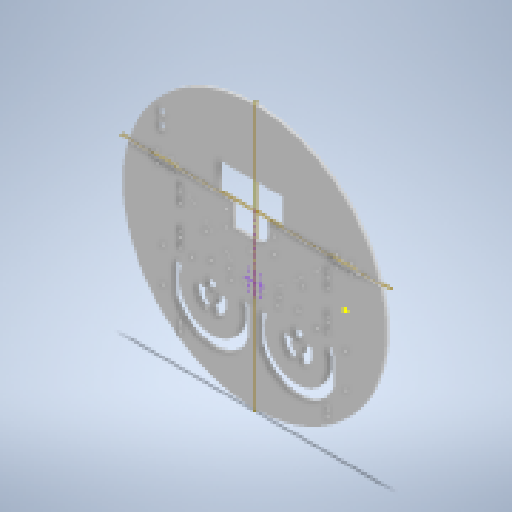
# Autodesk Inventor part: Деталь1
Saved by Autodesk Inventor 2023.2 (Build 272271030, 271C)
## iProperties
Created: 2024-01-26
Part Number: Деталь1
Material: Типовые
Document SubType Name: Modeling
Designer: I9232
Density: 1 g/cm^3
Appearance: По умолчанию
Author: I9232
Autodesk Inventor part; units mm, degrees
ref_plane "YZ Plane" through (0, 0, 0) normal (1, 0, 0) x (0, 1, 0)
ref_plane "XY Plane" through (0, 0, 0) normal (0, 0, 1) x (1, 0, 0)
sketch "Эскиз1" plane through (0, 0, 0) normal (0, 0, 1) x (1, 0, 0)
  circle A0 centre (-95.6307, 0) radius 137.5
  point P0 (0, 0)
  dimension "d61" = 275
  constraints: 1 centre point, 1 other
  measures "d61" diameter of A0
extrude "Выдавливание1" add sketch "Эскиз1" along normal blind 3
sketch "Эскиз5" plane through (0, 0, 3) normal (0, 0, 1) x (1, 0, 0)
  circle A0 centre (-191.4705, -72.9366) radius 1.5
  circle A1 centre (-191.4705, -37.0634) radius 1.5
  circle A2 centre (0, -37.0634) radius 1.5
  circle A3 centre (0, -72.9366) radius 1.5
  circle A4 centre (-30.8327, -32.3517) radius 1.5 projected
  circle A5 centre (-50.2499, -25.7302) radius 1.5 projected
  circle A6 centre (-70.9883, -32.7537) radius 1.5 projected
  circle A7 centre (-120.4823, -32.7537) radius 1.5 projected
  circle A8 centre (-141.2206, -25.7302) radius 1.5 projected
  circle A9 centre (-160.6378, -32.3517) radius 1.5 projected
  arc A10 (-12.7161, -49.3219) -> (-16.1637, -41.7649) centre (-51.5496, -62.4733) ccw projected
  line L0 (-12.7161, -49.3219) -> (-13.1664, -76.8861) projected
  arc A11 (-89.9328, -76.8861) -> (-13.1664, -76.8861) centre (-51.5496, -62.4733) ccw projected
  line L1 (-89.9328, -76.8861) -> (-90.3831, -49.3219) projected
  arc A12 (-88.8603, -45.4758) -> (-90.3831, -49.3219) centre (-51.5496, -62.4733) ccw projected
  line L2 (-88.8603, -45.4758) -> (-82.9355, -45.4758) projected
  arc A13 (-82.9355, -45.4758) -> (-20.1637, -46.3085) centre (-51.725, -59.1185) ccw projected
  line L3 (-20.1637, -46.3085) -> (-16.1637, -41.7649) projected
  line L4 (-178.9659, -76.8861) -> (-179.4162, -49.3219) projected
  arc A14 (-175.9686, -41.7649) -> (-179.4162, -49.3219) centre (-140.5827, -62.4733) ccw projected
  line L5 (-175.9686, -41.7649) -> (-171.9686, -46.3085) projected
  arc A15 (-171.9686, -46.3085) -> (-109.1968, -46.3085) centre (-140.5827, -59.1724) ccw projected
  line L6 (-109.1968, -46.3085) -> (-103.2721, -45.4758) projected
  arc A16 (-101.7492, -49.3219) -> (-103.2721, -45.4758) centre (-140.5827, -62.4733) ccw projected
  line L7 (-101.7492, -49.3219) -> (-102.1995, -76.8861) projected
  arc A17 (-178.9659, -76.8861) -> (-102.1995, -76.8861) centre (-140.5827, -62.4733) ccw projected
  arc A18 (-45.6461, -44.0105) -> (-55.6209, -44) centre (-50.6489, -58.6809) ccw projected
  line L8 (-45.6461, -44.0105) -> (-47.4855, -52.1853) projected
  arc A19 (-47.4855, -52.1853) -> (-53.8449, -52.3024) centre (-50.5504, -58.4786) ccw projected
  line L9 (-53.8449, -52.3024) -> (-55.6209, -44) projected
  line L10 (-135.8496, -44) -> (-137.6256, -52.3024) projected
  arc A20 (-137.6256, -52.3024) -> (-143.985, -52.1853) centre (-140.9201, -58.4786) ccw projected
  line L11 (-143.985, -52.1853) -> (-145.8244, -44.0105) projected
  arc A21 (-135.8496, -44) -> (-145.8244, -44.0105) centre (-140.8216, -58.6809) ccw projected
  arc A22 (-135.8665, -73.3675) -> (-126.822, -52.0281) centre (-140.8216, -58.6809) ccw projected
  line L12 (-135.8665, -73.3675) -> (-138.9215, -65.1872) projected
  arc A23 (-138.9215, -65.1872) -> (-135.0144, -54.7207) centre (-140.9201, -58.4786) ccw projected
  line L13 (-135.0144, -54.7207) -> (-126.822, -52.0281) projected
  arc A24 (-64.6485, -52.0281) -> (-55.604, -73.3675) centre (-50.6489, -58.6809) ccw projected
  line L14 (-64.6485, -52.0281) -> (-56.4561, -54.7207) projected
  arc A25 (-56.4561, -54.7207) -> (-52.549, -65.1872) centre (-50.5504, -58.4786) ccw projected
  line L15 (-52.549, -65.1872) -> (-55.604, -73.3675) projected
  arc A26 (-45.6939, -73.3676) -> (-36.6645, -51.9961) centre (-50.6489, -58.6809) ccw projected
  line L16 (-45.6939, -73.3676) -> (-48.7266, -65.2369) projected
  arc A27 (-48.7266, -65.2369) -> (-44.6776, -54.6694) centre (-50.5504, -58.4786) ccw projected
  line L17 (-44.6776, -54.6694) -> (-36.6645, -51.9961) projected
  arc A28 (-146.793, -54.6694) -> (-142.7439, -65.2369) centre (-140.9201, -58.4786) ccw projected
  line L18 (-142.7439, -65.2369) -> (-145.7766, -73.3676) projected
  arc A29 (-154.806, -51.9961) -> (-145.7766, -73.3676) centre (-140.8216, -58.6809) ccw projected
  line L19 (-154.806, -51.9961) -> (-146.793, -54.6694) projected
  dimension "d94" = 3
  dimension "d95" = 191.4705
  constraints: 4 centre point, 3 equal radius
  measures "d94" diameter of A3
  measures "d95" distance of A3.centre A0.centre
extrude "Выдавливание5" cut sketch "Эскиз5" against normal blind 3
sketch "Эскиз11" plane through (-95.6307, 0, 3) normal (0, 0, 1) x (1, 0, 0)
  line L0 (-6.5688, -36.8861) -> (-6.1185, -9.3219) construction
  line L1 (-6.3437, -23.104) -> (5.4727, -23.104) construction
  line L2 (5.6979, -36.8861) -> (5.2476, -9.3219) construction
  line L3 (-0.4355, 43.8357) -> (-0.4355, -36.6138) construction
  point P0 (95.6307, 0)
  point P1 (-0.4355, -23.104)
  constraints: 8 end point, 3 midpoint, 1 point on line, 1 vertical
ref_plane "Плоскость центральной симметрии" through (-96.0662, 43.8357, 3) normal (-1, 0, 0) x (0, -1, 0)
sketch "Эскиз8" plane through (0, 0, 3) normal (0, 0, 1) x (1, 0, 0)
  circle A0 centre (-197.0662, 34.25) radius 1.25
  circle A1 centre (-183.0662, 34.25) radius 1.25
  line L0 (-96.0662, -192.5) -> (-96.0662, 192.5) projected
  line L1 (-183.0662, 34.25) -> (-197.0662, 34.25) construction
  circle A2 centre (-183.0662, 44.75) radius 1.25
  circle A3 centre (-197.0662, 44.75) radius 1.25
  circle A4 centre (4.9338, 34.25) radius 1.25
  circle A5 centre (-9.0662, 34.25) radius 1.25
  line L2 (-9.0662, 34.25) -> (4.9338, 34.25) construction
  circle A6 centre (-9.0662, 44.75) radius 1.25
  circle A7 centre (4.9338, 44.75) radius 1.25
  line L3 (-183.0662, 34.25) -> (-183.0662, 44.75) construction
  line L4 (-183.0662, 39.5) -> (-192.8856, 39.5) construction
  line L5 (-197.0662, 44.75) -> (-197.0662, 34.25) construction
  point P0 (0, 0)
  dimension "d23" = 87
  dimension "d24" = 14
  dimension "d26" = 2.5
  dimension "d29" = 10.5
  dimension "d96" = 39.5
  constraints: 10 end point, 8 centre point, 4 symmetric about line, 3 vertical, 2 horizontal, 1 equal radius, 1 midpoint, 8 other
  measures "d23" distance from line of L1.start L0
  measures "d24" distance of L1.end L1.start
  measures "d26" diameter of A1
  measures "d29" distance of L1.start L3.end
  measures "d96" distance from line of L4 point (0, 0)
extrude "Выдавливание8" cut sketch "Эскиз8" against normal blind 3
sketch "Эскиз9" plane through (0, 0, 3) normal (0, 0, 1) x (1, 0, 0)
  point P0 (0, 0)
ref_plane "РабПлоскость2" through (0, 40, 0) normal (0, 1, 0) x (-1, 0, 0)
split body "Разделение2" result two bodies by plane through (0, 40, 0) normal (0, 1, 0) first body at (-95.921, 75.6667, 0.5)
sketch "Эскиз3" plane through (-95.6307, 0, 3) normal (0, 0, 1) x (1, 0, 0)
  circle A0 centre (0, 0) radius 137.5 projected
  line L0 (131.8531, 39) -> (-131.8531, 39)
  line L1 (131.245, 41) -> (-131.245, 41)
  arc A1 (-131.245, 41) -> (-131.8531, 39) centre (0, 0) ccw
  arc A2 (131.8531, 39) -> (131.245, 41) centre (9.2386, 2.8092) ccw
  line L2 (-192.5, 40) -> (192.5, 40) projected
  line L3 (-112.9264, 39) -> (-112.9264, 41) construction
  line L4 (131.5532, 40) -> (-131.5532, 40) projected
  point P0 (95.6307, 0)
  point P1 (-112.9264, 40)
  dimension "d63" = 2
  constraints: 8 point on circle, 6 end point, 3 point on line, 2 centre point, 1 concentric, 1 horizontal, 1 midpoint, 1 parallel, 1 perpendicular
  measures "d63" distance between parallel lines of L1 L0
extrude "Выдавливание3" cut sketch "Эскиз3" against normal blind 3 contours L0 A0 L2 | L2 A0 L1 bodies 2 3
sketch "Эскиз12" plane through (0, 0, 3) normal (0, 0, 1) x (1, 0, 0)
  line L0 (-171.3841, -10.2204) -> (-174.3841, -10.2204)
  line L1 (-174.3841, -10.2204) -> (-174.3841, -17.2204)
  line L2 (-174.3841, -17.2204) -> (-171.3841, -17.2204)
  line L3 (-171.3841, -17.2204) -> (-171.3841, -10.2204)
  line L4 (-171.3841, 15.777) -> (-174.3841, 15.777)
  line L5 (-174.3841, 15.777) -> (-174.3841, 8.777)
  line L6 (-174.3841, 8.777) -> (-171.3841, 8.777)
  line L7 (-171.3841, 8.777) -> (-171.3841, 15.777)
  line L8 (-171.3841, 29.777) -> (-174.3841, 29.777)
  line L9 (-174.3841, 29.777) -> (-174.3841, 22.777)
  line L10 (-174.3841, 22.777) -> (-171.3841, 22.777)
  line L11 (-171.3841, 22.777) -> (-171.3841, 29.777)
  line L12 (-174.3841, -108.1269) -> (-171.3841, -108.1269)
  line L13 (-171.3841, -108.1269) -> (-171.3841, -104.1269)
  line L14 (-171.3841, -104.1269) -> (-174.3841, -104.1269)
  line L15 (-174.3841, -104.1269) -> (-174.3841, -108.1269)
  line L16 (-174.3841, -99.1269) -> (-171.3841, -99.1269)
  line L17 (-171.3841, -99.1269) -> (-171.3841, -95.1269)
  line L18 (-171.3841, -95.1269) -> (-174.3841, -95.1269)
  line L19 (-174.3841, -95.1269) -> (-174.3841, -99.1269)
  line L20 (-96.0662, -192.5) -> (-96.0662, 192.5) construction
  line L21 (-171.3841, -24.2204) -> (-174.3841, -24.2204)
  line L22 (-174.3841, -24.2204) -> (-174.3841, -31.2204)
  line L23 (-174.3841, -31.2204) -> (-171.3841, -31.2204)
  line L24 (-171.3841, -31.2204) -> (-171.3841, -24.2204)
  line L25 (-20.7483, -10.2204) -> (-17.7483, -10.2204)
  line L26 (-17.7483, -10.2204) -> (-17.7483, -17.2204)
  line L27 (-17.7483, -17.2204) -> (-20.7483, -17.2204)
  line L28 (-20.7483, -17.2204) -> (-20.7483, -10.2204)
  line L29 (-20.7483, 15.777) -> (-17.7483, 15.777)
  line L30 (-17.7483, 15.777) -> (-17.7483, 8.777)
  line L31 (-17.7483, 8.777) -> (-20.7483, 8.777)
  line L32 (-20.7483, 8.777) -> (-20.7483, 15.777)
  line L33 (-20.7483, 29.777) -> (-17.7483, 29.777)
  line L34 (-17.7483, 29.777) -> (-17.7483, 22.777)
  line L35 (-17.7483, 22.777) -> (-20.7483, 22.777)
  line L36 (-20.7483, 22.777) -> (-20.7483, 29.777)
  line L37 (-17.7483, -108.1269) -> (-20.7483, -108.1269)
  line L38 (-20.7483, -108.1269) -> (-20.7483, -104.1269)
  line L39 (-20.7483, -104.1269) -> (-17.7483, -104.1269)
  line L40 (-17.7483, -104.1269) -> (-17.7483, -108.1269)
  line L41 (-17.7483, -99.1269) -> (-20.7483, -99.1269)
  line L42 (-20.7483, -99.1269) -> (-20.7483, -95.1269)
  line L43 (-20.7483, -95.1269) -> (-17.7483, -95.1269)
  line L44 (-17.7483, -95.1269) -> (-17.7483, -99.1269)
  line L45 (-20.7483, -24.2204) -> (-17.7483, -24.2204)
  line L46 (-17.7483, -24.2204) -> (-17.7483, -31.2204)
  line L47 (-17.7483, -31.2204) -> (-20.7483, -31.2204)
  line L48 (-20.7483, -31.2204) -> (-20.7483, -24.2204)
  circle A0 centre (-172.8841, -20.7204) radius 1.5
  circle A1 centre (-172.8841, -101.6269) radius 1.5
  circle A2 centre (-172.8841, 19.277) radius 1.5
  line L49 (-20.7483, -24.2204) -> (-17.7483, -24.2204)
  circle A3 centre (-19.2483, -20.7204) radius 1.5
  circle A4 centre (-19.2483, -101.6269) radius 1.5
  circle A5 centre (-19.2483, 19.277) radius 1.5
  point P0 (-172.8841, -99.1269)
  point P1 (-172.8841, -17.2204)
  point P2 (-172.8841, 22.777)
  dimension "d74" = 3
  dimension "d75" = 2.5
  dimension "d76" = 3.5
  dimension "d77" = 3.5
  constraints: 98 end point, 27 symmetric about line, 6 centre point, 3 midpoint, 2 equal radius, 3 other
  measures "d74" diameter of A0
  measures "d75" distance of point (-172.884, -99.127) A1.centre
  measures "d76" distance of point (-172.884, -17.22) A0.centre
  measures "d77" distance of point (-172.884, 22.777) A2.centre
extrude "Выдавливание10" cut sketch "Эскиз12" against normal through all bodies 3
sketch "Эскиз13" plane through (0, 0, 0) normal (0, 0, -1) x (-1, 0, 0)
  line L0 (196.3841, 65.7571) -> (190.3841, 65.7571) construction
  line L1 (190.3841, 65.7571) -> (190.3841, 85.7571) construction
  line L2 (190.3841, 85.7571) -> (196.3841, 85.7571) construction
  line L3 (196.3841, 85.7571) -> (196.3841, 65.7571) construction
  line L4 (196.3841, 65.7571) -> (190.3841, 65.7571)
  line L5 (190.3841, 65.7571) -> (190.3841, 72.7571)
  line L6 (190.3841, 72.7571) -> (196.3841, 72.7571)
  line L7 (196.3841, 72.7571) -> (196.3841, 65.7571)
  line L8 (196.3841, 75.7571) -> (190.3841, 75.7571) construction
  line L9 (196.3841, 85.7571) -> (190.3841, 85.7571) construction
  line L10 (196.3841, 85.7571) -> (190.3841, 85.7571)
  line L11 (190.3841, 85.7571) -> (190.3841, 78.7571)
  line L12 (190.3841, 78.7571) -> (196.3841, 78.7571)
  line L13 (196.3841, 78.7571) -> (196.3841, 85.7571)
  line L14 (149.3841, 76.0844) -> (149.3841, 68.5395) projected
  line L15 (193.3841, 78.7571) -> (193.3841, 72.7571) construction
  circle A0 centre (193.3841, 75.7571) radius 1.5
  line L16 (190.3841, 61.9127) -> (190.3841, 81.7469) projected
  point P0 (0, 0)
  point P1 (190.3841, 82.2571)
  dimension "d37" = 6
  dimension "d38" = 20
  dimension "d39" = 7
  dimension "d43" = 3
  dimension "d66" = 0
  constraints: 30 end point, 6 midpoint, 4 parallel, 4 symmetric about line, 2 horizontal, 2 perpendicular, 1 centre point, 1 point on line
  measures "d37" distance of L8.start L8.end
  measures "d38" distance of L2.end L0.start
  measures "d39" distance between parallel lines of L0 L6
  measures "d43" diameter of A0
  measures "d66" distance from line of L16 point (190.384, 82.257)
extrude "Выдавливание11" cut sketch "Эскиз13" against normal through all bodies 2
sketch "Эскиз16" plane through (0, 0, 3) normal (0, 0, 1) x (1, 0, 0)
  line L0 (-227.4838, 39) -> (36.2225, 39) projected
  line L1 (-96.0662, 39) -> (-96.0662, 41)
  line L2 (35.6143, 41) -> (-226.8757, 41) projected
  arc A0 (-96.0662, 15.3364) -> (-81.5178, 24.1698) centre (-94.6991, 29.482) ccw
  line L3 (-81.5178, 24.1698) -> (-81.5178, 39)
  line L4 (36.2225, 39) -> (-227.4838, 39) projected
  line L5 (-117.5429, 39) -> (-117.5429, 15.3364)
  arc A1 (-74.5894, 41) -> (-117.5429, 39) centre (-96.0662, 40) ccw
  line L6 (-96.0662, 15.3364) -> (-117.5429, 15.3364)
  point P0 (0, 0)
  point P1 (-117.5429, 41)
  constraints: 8 end point, 5 point on line, 4 point on circle, 3 perpendicular, 2 centre point, 1 midpoint
extrude "Выдавливание13" cut sketch "Эскиз16" against normal blind 3 contours L0 L3 A0 L6 L5 | A1 L2 bodies 2 3
sketch "Эскиз17" plane through (0, 0, 3) normal (0, 0, 1) x (1, 0, 0)
  circle A0 centre (-75.0461, 12) radius 1.25 projected
  circle A1 centre (-75.0662, 28.5) radius 1.25 projected
  circle A2 centre (-100.0461, 3.5) radius 1.25 projected
  circle A3 centre (-125.0461, 12) radius 1.25 projected
  circle A4 centre (-125.0662, 28.5) radius 1.25 projected
  point P0 (0, 0)
extrude "Выдавливание14" cut sketch "Эскиз17" against normal blind 3 bodies 3
sketch "Эскиз19" plane through (0, 0, 3) normal (0, 0, 1) x (1, 0, 0)
  circle A0 centre (-75.0461, 12) radius 1.25 projected
  circle A1 centre (-125.0461, 12) radius 1.25 projected
  circle A2 centre (-75.0662, 28.5) radius 1.25 projected
  circle A3 centre (-100.0461, 3.5) radius 1.25 projected
  circle A4 centre (-125.0662, 28.5) radius 1.25 projected
  arc A5 (-68.8662, 60) -> (-73.8662, 65) centre (-73.8662, 60) ccw projected
  arc A6 (-73.8662, -5) -> (-68.8662, 0) centre (-73.8662, 0) ccw projected
  line L0 (-73.8662, -5) -> (-124.2662, -5) projected
  line L1 (-131.2662, 2) -> (-131.2662, 60) projected
  arc A7 (-126.2662, 65) -> (-131.2662, 60) centre (-126.2662, 60) ccw projected
  line L2 (-126.2662, 65) -> (-108.2662, 65) projected
  line L3 (-116.2662, 50) -> (-116.2662, 21.4) projected
  line L4 (-108.2662, 10) -> (-83.8662, 10) projected
  line L5 (-83.8662, 10) -> (-83.8662, 60) projected
  arc A8 (-78.8662, 65) -> (-83.8662, 60) centre (-78.8662, 60) ccw projected
  line L6 (-78.8662, 65) -> (-73.8662, 65) projected
  line L7 (-74.5894, 41) -> (35.6143, 41) projected
  line L8 (-66.8662, 41) -> (-84.8662, 41)
  line L9 (-84.8662, 41) -> (-84.8662, 69)
  line L10 (-84.8662, 69) -> (-66.8662, 69)
  line L11 (-66.8662, 69) -> (-66.8662, 41)
  line L12 (-226.8757, 41) -> (-117.5429, 41) projected
  line L13 (-133.2662, 41) -> (-115.2662, 41)
  line L14 (-115.2662, 41) -> (-115.2662, 69)
  line L15 (-115.2662, 69) -> (-133.2662, 69)
  line L16 (-133.2662, 69) -> (-133.2662, 41)
  line L17 (-116.2662, 21.4) -> (-108.2662, 21.4) projected
  line L18 (-108.2662, 21.4) -> (-108.2662, 10) projected
  line L19 (-108.2662, 65) -> (-108.2662, 50) projected
  line L20 (-108.2662, 50) -> (-116.2662, 50) projected
  line L21 (-84.8662, 69) -> (-115.2662, 69)
  arc A9 (-131.2662, 2) -> (-124.2662, -5) centre (-124.2662, 2) ccw projected
  line L22 (-68.8662, 60) -> (-68.8662, 0) projected
  point P0 (0, 0)
  point P1 (-74.5894, 41)
  point P2 (-83.8662, 41)
  point P3 (-116.0662, 41)
  point P4 (-74.0662, 60)
  point P5 (-74.0662, 0)
  point P6 (-115.2662, 65)
  point P7 (-131.2662, 41)
  point P8 (-74.0662, 60)
  point P9 (-74.0662, 0)
  point P10 (-115.2662, 50)
  point P11 (-74.0662, 60)
  point P12 (-74.0662, 0)
  point P13 (-116.2662, 41)
  point P14 (-74.0662, 60)
  point P15 (-74.0662, 0)
  point P16 (-74.0662, 60)
  point P17 (-74.0662, 0)
  point P18 (-74.0662, 60)
  point P19 (-74.0662, 0)
  dimension "d53" = 28
  dimension "d54" = 28
  dimension "d57" = 1
  dimension "d58" = 1
  dimension "d64" = 18
  dimension "d65" = 18
  constraints: 18 end point, 4 parallel, 3 perpendicular, 3 point on line, 2 horizontal
  measures "d53" distance of L10.end L8.start
  measures "d54" distance of L15.end L13.start
  measures "d57" distance between parallel lines of L9 L5
  measures "d58" distance between parallel lines of L3 L14
  measures "d64" distance of L14.end L15.end
  measures "d65" distance of L9.end L10.end
extrude "Выдавливание15" cut sketch "Эскиз19" against normal blind 3 contours A0 | A1 | A2 | A3 | A4 | L22 L7 L8 L5 A8 L6 A5 | A5 L6 A8 L5 L8 L9 L10 L11 L7 L22 | L22 A6 L0 A9 L1 L12 L13 L3 L17 L18 L4 L5 L8 L7 | L5 L4 L18 L17 L3 L13 L14 L20 L19 L2 L21 L9 L8 | L14 L2 A7 L1 L12 L16 L15 | L14 L20 L3 L13 L12 L1 A7 L2 | L2 L19 L20 L14 | L14 L13 L3 L20 bodies 2
sketch "Эскиз20" plane through (0, 0, 3) normal (0, 0, 1) x (1, 0, 0)
  circle A0 centre (-147.1535, -2.0082) radius 1.45 projected
  circle A1 centre (-121.6186, -23.4345) radius 1.45 projected
  circle A2 centre (-96.0662, -40.2976) radius 1.45 projected
  circle A3 centre (-70.5137, -23.4345) radius 1.45 projected
  circle A4 centre (-44.9789, -2.0082) radius 1.45 projected
  point P0 (0, 0)
extrude "Выдавливание16" cut sketch "Эскиз20" against normal blind 3 bodies 2 3
sketch "Эскиз21" plane through (0, 0, 0) normal (0, 0, -1) x (-1, 0, 0)
  line L0 (147.5387, 7.4529) -> (137.5802, -0.9033) projected
  line L1 (147.5387, 7.4529) -> (147.3459, 7.6827) projected
  line L2 (147.3459, 7.6827) -> (137.3873, -0.6735) projected
  line L3 (137.5802, -0.9033) -> (137.3873, -0.6735) projected
  line L4 (166.8431, 23.6512) -> (156.8845, 15.2949) projected
  line L5 (166.8431, 23.6512) -> (166.6502, 23.881) projected
  line L6 (166.6502, 23.881) -> (156.6917, 15.5247) projected
  line L7 (156.8845, 15.2949) -> (156.6917, 15.5247) projected
  line L8 (128.2344, -8.7453) -> (118.2759, -17.1016) projected
  line L9 (128.2344, -8.7453) -> (128.0416, -8.5155) projected
  line L10 (128.0416, -8.5155) -> (118.083, -16.8718) projected
  line L11 (118.2759, -17.1016) -> (118.083, -16.8718) projected
  line L12 (108.9301, -24.9436) -> (98.9715, -33.2998) projected
  line L13 (108.9301, -24.9436) -> (108.7373, -24.7138) projected
  line L14 (108.7373, -24.7138) -> (98.7787, -33.07) projected
  line L15 (98.9715, -33.2998) -> (98.7787, -33.07) projected
  line L16 (83.2022, -24.9436) -> (93.1608, -33.2998) projected
  line L17 (93.1608, -33.2998) -> (93.3536, -33.07) projected
  line L18 (83.395, -24.7138) -> (93.3536, -33.07) projected
  line L19 (83.2022, -24.9436) -> (83.395, -24.7138) projected
  line L20 (63.8979, -8.7453) -> (73.8565, -17.1016) projected
  line L21 (73.8565, -17.1016) -> (74.0493, -16.8718) projected
  line L22 (64.0907, -8.5155) -> (74.0493, -16.8718) projected
  line L23 (63.8979, -8.7453) -> (64.0907, -8.5155) projected
  line L24 (44.5936, 7.4529) -> (54.5521, -0.9033) projected
  line L25 (54.5521, -0.9033) -> (54.745, -0.6735) projected
  line L26 (44.7864, 7.6827) -> (54.745, -0.6735) projected
  line L27 (44.5936, 7.4529) -> (44.7864, 7.6827) projected
  line L28 (25.2892, 23.6512) -> (35.2478, 15.2949) projected
  line L29 (35.2478, 15.2949) -> (35.4407, 15.5247) projected
  line L30 (25.4821, 23.881) -> (35.4407, 15.5247) projected
  line L31 (25.2892, 23.6512) -> (25.4821, 23.881) projected
  line L32 (21.459, 43.9586) -> (31.4176, 52.2964) projected
  line L33 (21.459, 43.9586) -> (21.6519, 43.7293) projected
  line L34 (21.6519, 43.7293) -> (31.6104, 52.0671) projected
  line L35 (31.4176, 52.2964) -> (31.6104, 52.0671) projected
  line L36 (40.7633, 60.1211) -> (50.7219, 68.459) projected
  line L37 (40.7633, 60.1211) -> (40.9562, 59.8918) projected
  line L38 (40.9562, 59.8918) -> (50.9148, 68.2297) projected
  line L39 (50.7219, 68.459) -> (50.9148, 68.2297) projected
  line L40 (60.0677, 76.2837) -> (70.0262, 84.6216) projected
  line L41 (60.0677, 76.2837) -> (60.2605, 76.0544) projected
  line L42 (60.2605, 76.0544) -> (70.2191, 84.3922) projected
  line L43 (70.0262, 84.6216) -> (70.2191, 84.3922) projected
  line L44 (79.372, 92.4463) -> (89.3306, 100.7841) projected
  line L45 (79.372, 92.4463) -> (79.5648, 92.217) projected
  line L46 (79.5648, 92.217) -> (89.5234, 100.5548) projected
  line L47 (89.3306, 100.7841) -> (89.5234, 100.5548) projected
  line L48 (112.7603, 92.4463) -> (102.8018, 100.7841) projected
  line L49 (102.8018, 100.7841) -> (102.6089, 100.5548) projected
  line L50 (112.5675, 92.217) -> (102.6089, 100.5548) projected
  line L51 (112.7603, 92.4463) -> (112.5675, 92.217) projected
  line L52 (132.0647, 76.2837) -> (122.1061, 84.6216) projected
  line L53 (122.1061, 84.6216) -> (121.9132, 84.3922) projected
  line L54 (131.8718, 76.0544) -> (121.9132, 84.3922) projected
  line L55 (132.0647, 76.2837) -> (131.8718, 76.0544) projected
  line L56 (151.369, 60.1211) -> (141.4104, 68.459) projected
  line L57 (141.4104, 68.459) -> (141.2176, 68.2297) projected
  line L58 (151.1761, 59.8918) -> (141.2176, 68.2297) projected
  line L59 (151.369, 60.1211) -> (151.1761, 59.8918) projected
  line L60 (170.6733, 43.9586) -> (160.7147, 52.2964) projected
  line L61 (160.7147, 52.2964) -> (160.5219, 52.0671) projected
  line L62 (170.4805, 43.7293) -> (160.5219, 52.0671) projected
  line L63 (170.6733, 43.9586) -> (170.4805, 43.7293) projected
  point P0 (0, 0)
extrude "Выдавливание17" cut sketch "Эскиз21" against normal blind 3 bodies 3
sketch "Эскиз25" plane through (0, 0, 3) normal (0, 0, 1) x (1, 0, 0)
  line L0 (-81.5178, 39) -> (36.2225, 39) projected
  line L1 (-17.0662, 39) -> (12.9338, 39)
  line L2 (12.9338, 39) -> (12.9338, 37)
  line L3 (12.9338, 37) -> (-17.0662, 37)
  line L4 (-17.0662, 37) -> (-17.0662, 39)
  line L5 (-66.8662, 41) -> (35.6143, 41) projected
  line L6 (-17.0662, 41) -> (12.9338, 41)
  line L7 (12.9338, 41) -> (12.9338, 43)
  line L8 (12.9338, 43) -> (-17.0662, 43)
  line L9 (-17.0662, 43) -> (-17.0662, 41)
  circle A0 centre (-9.0662, 34.25) radius 1.25 projected
  circle A1 centre (4.9338, 34.25) radius 1.25 projected
  line L10 (-9.0662, 34.25) -> (4.9338, 34.25)
  circle A2 centre (4.9338, 44.75) radius 1.25 projected
  circle A3 centre (-9.0662, 44.75) radius 1.25 projected
  line L11 (4.9338, 44.75) -> (-9.0662, 44.75)
  line L12 (-133.2662, 41) -> (-226.8757, 41) projected
  line L13 (-205.0662, 41) -> (-175.0662, 41)
  line L14 (-175.0662, 41) -> (-175.0662, 43)
  line L15 (-175.0662, 43) -> (-205.0662, 43)
  line L16 (-205.0662, 43) -> (-205.0662, 41)
  line L17 (-117.5429, 39) -> (-227.4838, 39) projected
  line L18 (-205.0662, 39) -> (-175.0662, 39)
  line L19 (-175.0662, 39) -> (-175.0662, 37)
  line L20 (-175.0662, 37) -> (-205.0662, 37)
  line L21 (-205.0662, 37) -> (-205.0662, 39)
  circle A4 centre (-183.0662, 44.75) radius 1.25 projected
  circle A5 centre (-197.0662, 44.75) radius 1.25 projected
  point P0 (0, 0)
  point P1 (-175.0662, 39)
  dimension "d78" = 30
  dimension "d79" = 2
  dimension "d80" = 2
  dimension "d82" = 30
  dimension "d86" = 30
  dimension "d87" = 2
  dimension "d88" = 2
  dimension "d89" = 30
  dimension "d91" = 8
  dimension "d93" = 8
  dimension "d97" = 8
  constraints: 36 end point, 8 parallel, 6 horizontal, 5 point on line, 4 perpendicular
  measures "d78" distance of L2.end L3.end
  measures "d79" distance of L1.end L2.end
  measures "d80" distance of L6.end L7.end
  measures "d82" distance of L7.end L8.end
  measures "d86" distance of L14.end L15.end
  measures "d87" distance of L13.end L14.end
  measures "d88" distance of L18.end L19.end
  measures "d89" distance of L19.end L20.end
  measures "d91" distance from line of L7 L11.start
  measures "d93" distance from line of A5.centre L16
  measures "d97" distance from line of L2 L10.end
extrude "Выдавливание19" cut sketch "Эскиз25" against normal blind 3 contours L0 L2 L3 L4 | L9 L8 L7 L5 | L12 L16 L15 L14 | L19 L20 L21 L17 bodies 3 2
mirror "Зеркальное отражение1" about plane through (-96.0662, 43.8357, 3) normal (-1, 0, 0) of "Выдавливание11" bodies 2
fillet "Сопряжение1" radius 3 4 edges at (-66.8662, 41, 1.5) (-133.2662, 41, 1.5) (-117.5429, 39, 1.5) (-81.5178, 39, 1.5)
fillet "Сопряжение2" radius 1 3 edges at (-66.8662, 69, 1.5) (-133.2662, 69, 1.5) (-117.5429, 15.3364, 1.5)
